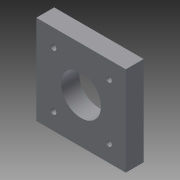
# Autodesk Inventor part: nema17gen
Saved by Autodesk Inventor 2014 SP2 (Build 180246200, 246)
## iProperties
Created: 2014-07-13
Part Number: nema17gen
Material: Generic
Document SubType Name: Modeling
Designer: cruiser
Density: 1 g/cm^3
Appearance: Default
Author: cruiser
Autodesk Inventor part; units mm, degrees
ref_plane "YZ Plane" through (0, 0, 0) normal (1, 0, 0) x (0, 1, 0)
ref_plane "XZ Plane" through (0, 0, 0) normal (0, 1, 0) x (-1, 0, 0)
ref_plane "XY Plane" through (0, 0, 0) normal (0, 0, 1) x (1, 0, 0)
sketch "Sketch1" plane through (0, 0, 0) normal (0, 1, 0) x (-1, 0, 0)
  line L0 (25, -25) -> (-25, -25)
  line L1 (-25, -25) -> (-25, 25)
  line L2 (-25, 25) -> (25, 25)
  line L3 (25, 25) -> (25, -25)
  line L4 (25, -25) -> (-25, 25) construction
  line L5 (-25, -25) -> (25, 25) construction
  point P0 (0, 0)
  dimension "d0" = 50
  dimension "d1" = 50
  constraints: 12 end point, 2 midpoint, 2 parallel, 1 horizontal, 1 perpendicular
  measures "d0" distance of L1.end L2.end
  measures "d1" distance of L0.end L1.end
extrude "Extrusion1" add sketch "Sketch1" along normal blind 10
sketch "Sketch7" plane through (0, 0, 0) normal (0, -1, 0) x (1, 0, 0)
  circle A0 centre (0, 0) radius 11.1
  line L0 (-15.5, -15.5) -> (15.5, -15.5)
  line L1 (15.5, -15.5) -> (15.5, 15.5)
  line L2 (15.5, 15.5) -> (-15.5, 15.5)
  line L3 (-15.5, 15.5) -> (-15.5, -15.5)
  line L4 (-15.5, -15.5) -> (15.5, 15.5) construction
  line L5 (15.5, -15.5) -> (-15.5, 15.5) construction
  circle A1 centre (-15.5, 15.5) radius 1.65
  circle A2 centre (-15.5, -15.5) radius 1.65
  circle A3 centre (15.5, -15.5) radius 1.65
  circle A4 centre (15.5, 15.5) radius 1.65
  dimension "d60" = 22.2
  dimension "d61" = 31
  dimension "d62" = 31
  dimension "d63" = 3.3
  dimension "d66" = 360
  constraints: 12 end point, 5 centre point, 2 coincident, 2 midpoint, 2 parallel, 1 horizontal, 1 perpendicular, 9 other
  measures "d60" diameter of A0
  measures "d61" distance of L2.end L1.end
  measures "d62" distance of L1.end L0.end
  measures "d63" diameter of A1
extrude "Extrusion6" cut sketch "Sketch7" against normal up to next contours A0 | L3 A2 L0 | L0 A2 L3 | A3 L1 L0 | L0 L1 A3 | A1 L2 L3 | L3 L2 A1 | A4 L2 L1 | L1 L2 A4
sketch "Sketch4" plane through (0, 0, 0) normal (0, -1, 0) x (1, 0, 0)
  line L0 (25, -25) -> (25, 25) projected
  line L1 (0, -22.2) -> (0, 22.2) construction
  line L2 (11.5, -22.2) -> (11.5, 22.2)
  line L3 (-11.5, 22.2) -> (-11.5, -22.2)
  arc A0 (-11.5, -22.2) -> (11.5, -22.2) centre (0, -22.2) ccw
  arc A1 (11.5, 22.2) -> (-11.5, 22.2) centre (0, 22.2) ccw
  line L4 (15.5, -15.5) -> (-15.5, -15.5)
  line L5 (-15.5, -15.5) -> (-15.5, 15.5)
  line L6 (-15.5, 15.5) -> (15.5, 15.5)
  line L7 (15.5, 15.5) -> (15.5, -15.5)
  line L8 (15.5, -15.5) -> (-15.5, 15.5) construction
  line L9 (-15.5, -15.5) -> (15.5, 15.5) construction
  line L10 (-15.5, -6.7) -> (-15.5, 37.7) construction
  line L11 (-13.85, -6.7) -> (-13.85, 37.7)
  line L12 (-17.15, 37.7) -> (-17.15, -6.7)
  arc A2 (-17.15, -6.7) -> (-13.85, -6.7) centre (-15.5, -6.7) ccw
  arc A3 (-13.85, 37.7) -> (-17.15, 37.7) centre (-15.5, 37.7) ccw
  line L13 (15.5, -6.7) -> (15.5, 37.7) construction
  line L14 (17.15, -6.7) -> (17.15, 37.7)
  line L15 (13.85, 37.7) -> (13.85, -6.7)
  arc A4 (13.85, -6.7) -> (17.15, -6.7) centre (15.5, -6.7) ccw
  arc A5 (17.15, 37.7) -> (13.85, 37.7) centre (15.5, 37.7) ccw
  line L16 (-15.5, -37.7) -> (-15.5, 6.7) construction
  line L17 (-13.85, -37.7) -> (-13.85, 6.7)
  line L18 (-17.15, 6.7) -> (-17.15, -37.7)
  arc A6 (-17.15, -37.7) -> (-13.85, -37.7) centre (-15.5, -37.7) ccw
  arc A7 (-13.85, 6.7) -> (-17.15, 6.7) centre (-15.5, 6.7) ccw
  line L19 (15.5, -37.7) -> (15.5, 6.7) construction
  line L20 (17.15, -37.7) -> (17.15, 6.7)
  line L21 (13.85, 6.7) -> (13.85, -37.7)
  arc A8 (13.85, -37.7) -> (17.15, -37.7) centre (15.5, -37.7) ccw
  arc A9 (17.15, 6.7) -> (13.85, 6.7) centre (15.5, 6.7) ccw
  line L22 (25, -25) -> (-25, -25)
  line L23 (-25, -25) -> (-25, 25)
  line L24 (-25, 25) -> (25, 25)
  line L25 (25, 25) -> (25, -25)
  line L26 (25, -25) -> (-25, 25) construction
  line L27 (-25, -25) -> (25, 25) construction
  line L28 (0, 0) -> (0, 25)
  line L29 (0, 0) -> (-25, 0)
  line L30 (0, 0) -> (25, 0)
  line L31 (0, 0) -> (0, -25)
  dimension "d25" = 22.2
  dimension "d26" = 23
  dimension "d27" = 31
  dimension "d28" = 31
  dimension "d29" = 22.2
  dimension "d30" = 3.3
  dimension "d31" = 22.2
  dimension "d32" = 3.3
  dimension "d33" = 22.2
  dimension "d34" = 3.3
  dimension "d35" = 22.2
  dimension "d36" = 3.3
  constraints: 72 end point, 20 point on circle, 20 tangent, 15 midpoint, 11 parallel, 10 centre point, 3 perpendicular, 2 horizontal, 2 point on line
  measures "d25" distance of L28.start L1.end
  measures "d26" distance between parallel lines of L2 L3
  measures "d27" distance of L5.end L6.end
  measures "d28" distance of L4.end L5.end
  measures "d29" distance of L5.end L10.end
  measures "d30" diameter of A3
  measures "d31" distance of L6.end L13.end
  measures "d32" diameter of A5
  measures "d33" distance of L4.end L16.end
  measures "d34" diameter of A7
  measures "d35" distance of L4.start L19.end
  measures "d36" diameter of A9
equation "\"d60\" = center_hole"
equation "\"d63\" = mount_hole"
equation "\"d25\" = center_hole"
equation "\"d29\" = center_hole"
equation "\"d31\" = center_hole"
equation "\"d33\" = center_hole"
equation "\"d35\" = center_hole"
equation "\"center_hole\" = 22.2"
equation "\"mount_hole\" = 3.3"
body "Solid1"
